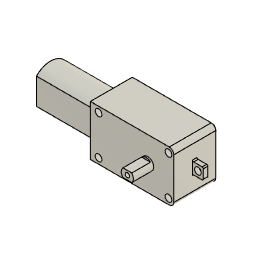
TTMotorOld v1 (Autodesk Fusion 360 design; units mm, degrees)
Autodesk Fusion 360 part; units mm, degrees
sketch "Sketch1" plane through (0, 0, 0) normal (0, 0, 1) x (1, 0, 0)
  line L0 (-2, 0) -> (-64, 0)
  line L1 (-64, 0) -> (-64, 22.3)
  line L2 (-64, 22.3) -> (-2, 22.3)
  line L3 (0, 20.3) -> (0, 2)
  line L4 (-37, 22.3) -> (-37, 0)
  line L5 (0, 13.65) -> (4.8, 13.65)
  line L6 (4.8, 13.65) -> (4.8, 8.65)
  line L7 (4.8, 8.65) -> (0, 8.65)
  line L8 (0, 8.65) -> (0, 13.65)
  circle A0 centre (2.4, 11.15) radius 1.5
  line L9 (-11.6, 22.3) -> (-11.6, 0) construction
  circle A1 centre (-11.6, 11.15) radius 2.7
  circle A2 centre (-2.35, 19.815) radius 1.5
  circle A3 centre (-2.35, 2.485) radius 1.5
  line L10 (-2.35, 19.815) -> (-2.35, 22.3) construction
  line L11 (-2.35, 2.485) -> (-2.35, 0) construction
  arc A4 (0, 20.3) -> (-2, 22.3) centre (-2, 20.3) ccw
  arc A5 (-2, 0) -> (0, 2) centre (-2, 2) ccw
  line L12 (-13.5666, 13) -> (-9.6334, 13)
  line L13 (-13.5666, 9.3) -> (-9.6334, 9.3)
  circle A6 centre (-11.6, 11.15) radius 0.975
  line L14 (-37, 17.515) -> (-64, 17.515)
  line L15 (-37, 4.785) -> (-64, 4.785)
  line L16 (-53.8571, 22.3) -> (-53.8571, 17.515) construction
  line L17 (-53.8571, 4.785) -> (-53.8571, 0) construction
  line L18 (-11.6, 11.15) -> (-22.85, 11.15) construction
  circle A7 centre (-22.85, 11.15) radius 2
  circle A8 centre (-33.35, 2.485) radius 1.5
  circle A9 centre (-33.35, 19.815) radius 1.5
  point P0 (0, 22.3)
  point P1 (0, 11.15)
  dimension "d1" = 64
  dimension "d2" = 22.3
  dimension "d3" = 37
  dimension "d4" = 4.8
  dimension "d5" = 5
  dimension "d6" = 3
  dimension "d7" = 14
  dimension "d8" = 5.4
  dimension "d9" = 17.33
  dimension "d10" = 9.25
  dimension "d11" = 2
  dimension "d12" = 2
  dimension "d13" = 3.7
  dimension "d14" = 1.95
  dimension "d15" = 12.73
  dimension "d16" = 11.25
  dimension "d17" = 4
  dimension "d18" = 3
  dimension "d19" = 3
  dimension "d20" = 17.33
  dimension "d21" = 3
  dimension "d22" = 3
  dimension "d29" = 11.15
  constraint horizontal L0
  constraint vertical L1
  constraint horizontal L2
  constraint vertical L3
  constraint coincident L2 L4.start
  constraint coincident L0 L4.end
  constraint perpendicular L0 L4
  constraint horizontal L5
  constraint vertical L6
  constraint horizontal L7
  constraint vertical L8
  constraint midpoint L8 P1
  constraint coincident L2 L9.start
  constraint perpendicular L2 L9
  constraint coincident L9 A1.centre
  constraint coincident A2.centre L10.start
  constraint coincident L2 L10.end
  constraint perpendicular L2 L10
  constraint coincident A3.centre L11.start
  constraint coincident L0 L11.end
  constraint perpendicular L0 L11
  constraint equal L10 L11
  constraint collinear L10 L11
  constraint coincident L3 P1
  constraint coincident P0 L2
  constraint coincident P0 L3
  constraint tangent L2 A4
  constraint tangent L3 A4
  constraint coincident origin L0
  constraint coincident origin L3
  constraint tangent L0 A5
  constraint tangent L3 A5
  constraint coincident A1 L12.start
  constraint coincident A1 L12.end
  constraint perpendicular L9 L12
  constraint coincident A1 L13.start
  constraint coincident A1 L13.end
  constraint perpendicular L9 L13
  constraint equal L12 L13
  constraint concentric A1 A6
  constraint coincident L4 L14.start
  constraint coincident L1 L14.end
  constraint perpendicular L1 L14
  constraint coincident L4 L15.start
  constraint coincident L1 L15.end
  constraint perpendicular L1 L15
  constraint coincident L2 L16.start
  constraint coincident L14 L16.end
  constraint perpendicular L14 L16
  constraint coincident L15 L17.start
  constraint coincident L0 L17.end
  constraint perpendicular L0 L17
  constraint equal L16 L17
  constraint coincident A1.centre A6.centre
  constraint perpendicular L9 L18
  constraint coincident L18.end A7.centre
  measures "d1" distance of origin L0.end
  measures "d2" distance of origin P0
  measures "d3" distance of L3 L4
  measures "d4" distance of L5.start L5.end
  measures "d5" distance of L5.start L7.end
  measures "d6" diameter of A0
  measures "d7" distance of A0.centre L9
  measures "d8" diameter of A1
  measures "d9" distance of A2.centre A3.centre
  measures "d10" distance of L9 L10
  measures "d11" radius of A4
  measures "d12" radius of A5
  measures "d13" distance of L12 L13
  measures "d14" diameter of A6
  measures "d15" distance of L14 L15
  measures "d16" distance of A1.centre L18.end
  measures "d17" diameter of A7
  measures "d18" diameter of A2
  measures "d19" diameter of A3
  measures "d20" distance of A8.centre A9.centre
  measures "d21" diameter of A9
  measures "d22" diameter of A8
  measures "d29" distance of L0 L18
extrude "Extrude1" add sketch "Sketch1" along normal mid plane 18.6 contours L0 L2 L3 L4 L8 A4 A5
extrude "Extrude2" add sketch "Sketch1" along normal mid plane 20 contours A1 L12 | A1 L13
extrude "Extrude3" add sketch "Sketch1" along normal mid plane 36.6 contours A1 L12 L13
sketch "Sketch2" plane through (-37, 0, 0) normal (-1, 0, 0) x (0, -1, 0)
  line L0 (0, -9.3) -> (0, 9.3)
  line L1 (0, 9.3) -> (-22.3, 9.3)
  line L2 (-22.3, 9.3) -> (-22.3, -9.3)
  line L3 (-22.3, -9.3) -> (0, -9.3)
  line L4 (0, 0) -> (-22.3, 0)
  circle A0 centre (-11.15, 0) radius 8.5
  line L5 (-16.9646, 6.2) -> (-5.3354, 6.2)
  line L6 (-16.9646, -6.2) -> (-5.3354, -6.2)
  dimension "d30" = 17
  dimension "d31" = 6.2
  constraint midpoint L4 A0.centre
  constraint coincident A0 L5.start
  constraint coincident A0 L5.end
  constraint parallel L4 L5
  constraint symmetric L4 L5.start L6.start
  constraint symmetric L4 L5.end L6.end
  measures "d30" diameter of A0
  measures "d31" distance of L4 L5
extrude "Extrude4" add sketch "Sketch2" along normal blind 27 contours L4 A0 L6 | L4 A0 L5
extrude "Extrude5" add sketch "Sketch1" along normal mid plane 2 contours L3 L5 L6 L7 L8
extrude "Extrude6" add sketch "Sketch1" along normal blind 11.22 contours A7
extrude "Extrude7" add sketch "Sketch1" against normal blind 9.3 contours A7
fillet "Fillet1" radius 0.5 4 edges at (0, 13.65, 0) (0, 8.65, 0) (4.8, 8.65, 0) (4.8, 13.65, 0)
move_body "Move1" bodies 1 to x (1, 0, 0) y (0, 0, -1) z (0, 1, 0) at (0, 18.3, -18.3)
move_body "Move2" bodies 1 to x (1, 0, 0) y (0, 1, 0) z (0, 0, 1) at (37, -18.3, 29.45)
equation "d23 = ( 18.6 / 2 ) * 1 mm"
equation "d36 = 9.30 mm + 1.92 mm"
